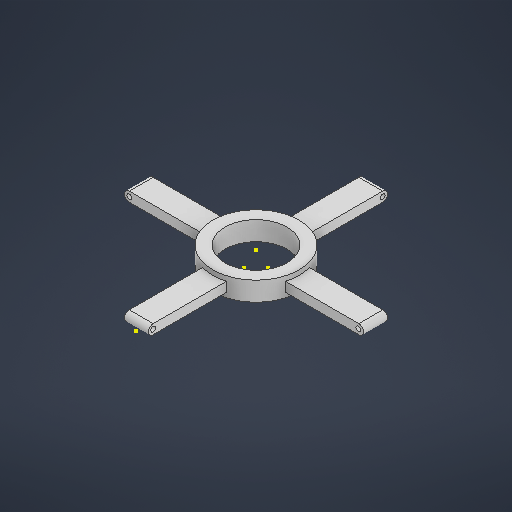
# Autodesk Inventor part: Pieza6
Saved by Autodesk Inventor 2026.1 (Build 301233000, 233)
## iProperties
Created: 2025-09-19
Part Number: Pieza6
Material: Genérico
Document SubType Name: Modeling
Designer: Usuario
Density: 1 g/cm^3
Appearance: Valor por defecto
Author: Usuario
Autodesk Inventor part; units mm, degrees
ref_plane "YZ Plane" through (0, 0, 0) normal (1, 0, 0) x (0, 1, 0)
ref_plane "XZ Plane" through (0, 0, 0) normal (0, 1, 0) x (-1, 0, 0)
ref_plane "XY Plane" through (0, 0, 0) normal (0, 0, 1) x (1, 0, 0)
sketch "Boceto1" plane through (0, 0, 0) normal (0, 1, 0) x (-1, 0, 0)
  circle A0 centre (0, 0) radius 50 construction
  line L0 (-28.7316, 0) -> (21.6034, 0) construction
  circle A1 centre (0, 0) radius 12.95
  line L1 (50, 0) -> (-50, 0) construction
  line L2 (-50, 0) -> (-50, 5)
  line L3 (50, 5) -> (50, 0)
  line L4 (-50, 0) -> (-50, -5)
  line L5 (50, -5) -> (50, 0)
  line L6 (-50, -5) -> (-17.2916, -5)
  line L7 (17.2916, -5) -> (50, -5)
  line L8 (-50, 5) -> (-17.2916, 5)
  line L9 (17.2916, 5) -> (50, 5)
  line L10 (0, 50) -> (0, -50) construction
  line L11 (0, -50) -> (-5, -50)
  line L12 (-5, 50) -> (0, 50)
  line L13 (0, -50) -> (5, -50)
  line L14 (5, 50) -> (0, 50)
  arc A2 (-17.2916, -5) -> (-5, -17.2916) centre (0, 0) ccw
  arc A3 (5, -17.2916) -> (17.2916, -5) centre (0, 0) ccw
  arc A4 (17.2916, 5) -> (5, 17.2916) centre (0, 0) ccw
  arc A5 (-5, 17.2916) -> (-17.2916, 5) centre (0, 0) ccw
  line L15 (-5, -50) -> (-5, -17.2916)
  line L16 (-5, 17.2916) -> (-5, 50)
  line L17 (5, 17.2916) -> (5, 50)
  line L18 (5, -50) -> (5, -17.2916)
  dimension "d2" = 100
  dimension "d3" = 25.9
  dimension "d5" = 5
  dimension "d6" = 5
  constraints: 38 end point, 12 point on circle, 6 centre point, 6 parallel, 4 symmetric about line, 2 coincident, 2 horizontal, 2 perpendicular, 1 vertical
  measures "d2" diameter of A0
  measures "d3" diameter of A1
  measures "d5" distance of L1.end L2.end
  measures "d6" distance of L10.end L11.end
extrude "Extrusión1" add sketch "Boceto1" along normal blind 4
sketch "Boceto2" plane through (0, 4, 0) normal (0, 1, 0) x (1, 0, 0)
  circle A0 centre (0, 0) radius 18
  circle A1 centre (0, 0) radius 12.95
  dimension "d9" = 36
  dimension "d10" = 25.9
  constraints: 2 centre point, 2 coincident
  measures "d9" diameter of A0
  measures "d10" diameter of A1
extrude "Extrusión2" add sketch "Boceto2" along normal blind 2
sketch "Boceto3" plane through (0, 0, 0) normal (0, -1, 0) x (1, 0, 0)
  circle A0 centre (0, 0) radius 18
  circle A1 centre (0, 0) radius 12.95
  dimension "d13" = 36
  dimension "d14" = 25.9
  constraints: 2 centre point, 2 coincident
  measures "d13" diameter of A0
  measures "d14" diameter of A1
extrude "Extrusión3" add sketch "Boceto3" along normal blind 2
sketch "Boceto4" plane through (0, 4, 0) normal (0, 1, 0) x (1, 0, 0)
  point P0 (0, 0)
sketch "Boceto5" plane through (-5, 0, 50) normal (0, 0, 1) x (1, 0, 0)
  point P0 (5, 0)
sketch "Boceto6" plane through (-5, 0, 17.2916) normal (-1, 0, 0) x (0, 0, 1)
  line L0 (-67.2916, 4) -> (-63.2916, 4) construction
  line L1 (-63.2916, 4) -> (-63.2916, 0) construction
  line L2 (-63.2916, 0) -> (-67.2916, 0) construction
  line L3 (-67.2916, 0) -> (-67.2916, 4) construction
  line L4 (32.7084, 4) -> (0, 4) construction
  line L5 (32.7084, 4) -> (28.7084, 4)
  line L6 (28.7084, 4) -> (28.7084, 0) construction
  line L7 (28.7084, 0) -> (32.7084, 0) construction
  line L8 (32.7084, 0) -> (32.7084, 4) construction
  circle A0 centre (30.7084, 2) radius 1
  circle A1 centre (-65.2916, 2) radius 1
  point P0 (-17.2916, 0)
  dimension "d17" = 4
  dimension "d18" = 4
  dimension "d19" = 4
  dimension "d20" = 4
  dimension "d21" = 2
  dimension "d22" = 2
  constraints: 16 end point, 4 parallel, 2 centre point, 2 horizontal, 2 perpendicular
  measures "d17" distance of L1.end L2.end
  measures "d18" distance of L0.end L1.end
  measures "d19" distance of L7.end L6.end
  measures "d20" distance of L6.end L5.end
  measures "d21" diameter of A0
  measures "d22" diameter of A1
extrude "Extrusión4" cut sketch "Boceto6" against normal through all
sketch "Boceto7" plane through (17.2916, 0, 5) normal (0, 0, 1) x (1, 0, 0)
  line L0 (-34.5832, 4) -> (-67.2916, 4) construction
  line L1 (-67.2916, 4) -> (-63.2916, 4)
  line L2 (-63.2916, 4) -> (-63.2916, 0) construction
  line L3 (-63.2916, 0) -> (-67.2916, 0) construction
  line L4 (-67.2916, 0) -> (-67.2916, 4) construction
  circle A0 centre (-65.2916, 2) radius 1
  line L5 (32.7084, 4) -> (0, 4) construction
  line L6 (32.7084, 4) -> (28.7084, 4)
  line L7 (28.7084, 4) -> (28.7084, 0) construction
  line L8 (28.7084, 0) -> (32.7084, 0) construction
  line L9 (32.7084, 0) -> (32.7084, 4) construction
  circle A1 centre (30.5299, 2) radius 1
  point P0 (-17.2916, 0)
  dimension "d25" = 4
  dimension "d26" = 4
  dimension "d27" = 2
  dimension "d28" = 4
  dimension "d29" = 4
  dimension "d30" = 2
  constraints: 16 end point, 4 parallel, 2 centre point, 2 horizontal, 2 perpendicular
  measures "d25" distance of L2.end L3.end
  measures "d26" distance of L1.end L2.end
  measures "d27" diameter of A0
  measures "d28" distance of L8.end L7.end
  measures "d29" distance of L7.end L6.end
  measures "d30" diameter of A1
extrude "Extrusión5" cut sketch "Boceto7" against normal through all
fillet "Empalme1" radius 2 8 edges at (-50, 4, 0) (-50, 0, 0) (0, 4, 50) (0, 0, 50) (50, 4, 0) (50, 0, 0) (0, 4, -50) (0, 0, -50)
sketch "Boceto8" plane through (-17.2916, 0, 5) normal (0, 0, 1) x (1, 0, 0)
  point P0 (17.2916, 0)
sketch "Boceto9" plane through (5, 0, 17.2916) normal (1, 0, 0) x (0, 0, -1)
  point P0 (17.2916, 0)
